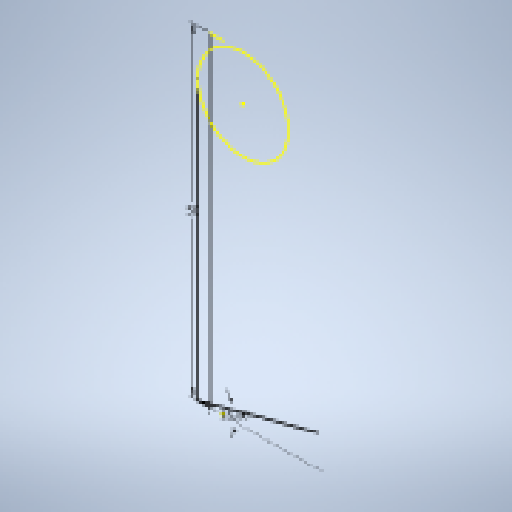
# Autodesk Inventor part: noz
Saved by Autodesk Inventor 2023 (Build 270158000, 158)
## iProperties
Created: 2023-12-19
Part Number: noz
Material: Ogólny
Document SubType Name: Modeling
Designer: Kamil
Density: 1 g/cm^3
Appearance: Domyślna
Author: Kamil
Autodesk Inventor part; units mm, degrees
ref_plane "YZ Plane" through (0, 0, 0) normal (1, 0, 0) x (0, 1, 0)
ref_plane "XZ Plane" through (0, 0, 0) normal (0, 1, 0) x (-1, 0, 0)
ref_plane "XY Plane" through (0, 0, 0) normal (0, 0, 1) x (1, 0, 0)
sketch "Szkic1" plane through (0, 0, 0) normal (0, 0, 1) x (1, 0, 0)
  circle A0 centre (3.1, 43) radius 7 projected
  line L0 (-2, 50) -> (-2, 0)
  line L1 (-2, 50) -> (0, 50) projected
  line L2 (-3.9, 43) -> (-3.9, 0)
  line L3 (-3.9, 0) -> (-2, 0)
  line L4 (-3.9, 0) -> (14.8489, 5.0238)
  line L5 (-3.9, 0) -> (15.5103, 0) construction
  line L6 (1.3909, 1.4177) -> (0.8733, 3.3496)
  line L7 (0.8733, 3.3496) -> (-3.9, 2.0706)
  line L8 (0.8733, 3.3496) -> (13.2644, 6.6697)
  line L9 (13.85, 30) -> (13.85, 0) projected
  line L10 (13.85, 6.8267) -> (16.85, 7.6305)
  line L11 (13.85, 4.7561) -> (16.85, 5.5599)
  line L12 (16.85, 7.6305) -> (16.85, 5.5599)
  line L13 (13.85, 6.8267) -> (13.2644, 6.6697)
  point P0 (0, 0)
  point P1 (-2, 0)
  point P2 (16.85, 6.5952)
  dimension "d0" = 50
  dimension "d1" = 15
  dimension "d2" = 2
  dimension "d3" = 3
  constraints: 24 end point, 8 point on line, 4 parallel, 3 vertical, 2 perpendicular, 1 collinear, 1 equal length, 1 horizontal, 1 horizontal alignment, 1 midpoint, 2 other
  measures "d0" distance of L0.start L0.end
  measures "d1" angle of L5 L4
  measures "d2" distance of L6.start L6.end
  measures "d3" distance from line of L9 point (16.85, 6.595)
extrude "Wyciągnięcie proste1" add sketch "Szkic1" against normal blind 50 contours L7 L6 L4 L0 | L0 L4 L2 L7 | L8 L13 L9 L4 L6 | L9 L10 L12 L11 L4
